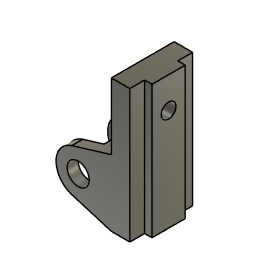
Sectional_Views_Model_Sliding_Block (Autodesk Fusion 360 design; units mm, degrees)
Autodesk Fusion 360 part; units mm, degrees
sketch "Sketch1" plane through (0, 0, 0) normal (0, 1, 0) x (1, 0, 0)
  circle A0 centre (0, 0) radius 15
  line L0 (45, 45) -> (70, 45)
  line L1 (45, -45) -> (45, -135)
  line L2 (45, -135) -> (70, -135)
  line L3 (70, -135) -> (70, 0)
  line L4 (70, 0) -> (70, 45)
  line L5 (45, -135) -> (45, -45)
  line L6 (45, -45) -> (-8.7083, -28.7083)
  line L7 (45, 45) -> (-11.6322, 27.8214)
  line L8 (0, -30) -> (0, -31.3498)
  arc A1 (-8.7083, 28.7083) -> (-8.7083, -28.7083) centre (0, 0) ccw
  dimension "d1" = 60
  dimension "d2" = 30
  dimension "d3" = 70
  dimension "d5" = 25
  dimension "d6" = 180
  constraint coincident A0.centre A1.centre
  constraint concentric A0 A1
  constraint perpendicular L0 L1
  constraint perpendicular L1 L2
  constraint perpendicular L0 L4
  constraint tangent L6 A1
  constraint tangent L7 A1
  constraint coincident L6 L8.end
  constraint coincident L7 A1.start
  measures "d1" diameter of A1
  measures "d2" diameter of A0
  measures "d3" distance of A0.centre L3.end
  measures "d5" distance of L0.end L0.start
  measures "d6" distance of L0.start L1.end
extrude "Extrude1" add sketch "Sketch1" along normal blind 85
sketch "Sketch2" plane through (45, 0, 0) normal (-1, 0, 0) x (0, -1, 0)
  line L0 (0, 45) -> (0, 135)
  line L1 (0, 135) -> (-85, 135)
  line L2 (-85, 135) -> (-85, 45)
  line L3 (-85, 45) -> (0, 45)
sketch "Sketch3" plane through (70, 0, 0) normal (1, 0, 0) x (0, 1, 0)
  line L0 (0, 135) -> (0, -45)
  line L1 (0, -45) -> (85, -45)
  line L2 (85, -45) -> (85, 135)
  line L3 (85, 135) -> (0, 135)
  line L4 (85, -45.5194) -> (85, -45)
  constraint vertical L4
sketch "Sketch4" plane through (70, 0, 0) normal (1, 0, 0) x (0, 1, 0)
  line L0 (20, 135) -> (20, -45)
  line L1 (20, -45) -> (65, -45)
  line L2 (65, -45) -> (65, 135)
  line L3 (65, 135) -> (20, 135)
  constraint vertical L0
  constraint perpendicular L0 L1
  constraint perpendicular L1 L2
  constraint perpendicular L0 L3
extrude "Extrude2" add sketch "Sketch4" along normal blind 10
sketch "Sketch5" plane through (45, 0, 0) normal (-1, 0, 0) x (0, -1, 0)
ref_plane "WorkPlane1" through (45, 0, 135) normal (-1, 0, 0) x (0, -1, 0)
sketch "Sketch6" plane through (45, 0, 0) normal (-1, 0, 0) x (0, -1, 0)
sketch "Sketch7" plane through (45, 0, 0) normal (-1, 0, 0) x (0, -1, 0)
  circle A0 centre (-42.5, 93) radius 25
  dimension "d18" = 50
  measures "d18" diameter of A0
sketch "Sketch8" plane through (45, 0, 0) normal (-1, 0, 0) x (0, -1, 0)
sketch "Sketch9" plane through (45, 0, 0) normal (-1, 0, 0) x (0, -1, 0)
sketch "Sketch10" plane through (45, 0, 0) normal (-1, 0, 0) x (0, -1, 0)
  circle A0 centre (-42.5, 93) radius 10
  dimension "d21" = 20
  measures "d21" diameter of A0
extrude "Extrude3" cut sketch "Sketch10" against normal blind 70
extrude "Extrude4" cut sketch "Sketch7" against normal blind 10
ref_plane "WorkPlane2" through (45, 0, 45) normal (-0.290276, 0, 0.956943) x (0, -1, 0)
sketch "Sketch11" plane through (-8.7083, 0, 28.7083) normal (-0.290276, 0, 0.956943) x (0, -1, 0)
sketch "Sketch12" plane through (0, 0, 0) normal (0, -1, 0) x (1, 0, 0)
  circle A0 centre (0, 0) radius 15
  line L0 (-8.7083, -28.7083) -> (45, -45)
  line L1 (45, -45) -> (70, -45)
  line L2 (70, -45) -> (70, 135)
  line L3 (70, 135) -> (45, 135)
  line L4 (45, 135) -> (45, 45)
  line L5 (45, 45) -> (-8.7083, 28.7083)
  arc A1 (-8.7083, 28.7083) -> (-8.7083, -28.7083) centre (0, 0) ccw
sketch "Sketch13" plane through (70, 0, 0) normal (1, 0, 0) x (0, 1, 0)
sketch "Sketch14" plane through (0, 0, 0) normal (0, -1, 0) x (1, 0, 0)
ref_plane "WorkPlane3" through (45, 0, -45) normal (0, -1, 0) x (1, 0, 0)
sketch "Sketch15" plane through (0, 0, 0) normal (0, -1, 0) x (-1, 0, 0)
ref_plane "WorkPlane4" through (45, 85, -45) normal (0, 1, 0) x (-1, 0, 0)
sketch "Sketch16" plane through (0, 85, 0) normal (0, 1, 0) x (1, 0, 0)
sketch "Sketch17" plane through (-8.7083, 0, 28.7083) normal (-0.290276, 0, 0.956943) x (0, -1, 0)
  line L0 (0, 0) -> (0, 56.1249)
  line L1 (0, 56.1249) -> (-85, 56.1249)
  line L2 (-85, 56.1249) -> (-85, 0)
sketch "Sketch18" plane through (45, 0, 0) normal (-1, 0, 0) x (0, -1, 0)
  line L0 (-85, 45) -> (0, 45)
  line L1 (0, 45) -> (0, 50)
  line L2 (0, 50) -> (-85, 50)
  line L3 (-85, 50) -> (-85, 45)
  constraint horizontal L0
  constraint perpendicular L0 L1
  constraint perpendicular L1 L2
  constraint perpendicular L0 L3
extrude "Extrude5" add sketch "Sketch18" along normal blind 200
sketch "Sketch19" plane through (0, 0, 0) normal (0, -1, 0) x (1, 0, 0)
ref_plane "WorkPlane5" through (-155, 0, 45) normal (0, 0, -1) x (-1, 0, 0)
sketch "Sketch20" plane through (0, 0, 45) normal (0, 0, -1) x (-1, 0, 0)
sketch "Sketch21" plane through (0, 0, 0) normal (0, -1, 0) x (1, 0, 0)
sketch "Sketch22" plane through (0, 85, 0) normal (0, 1, 0) x (-1, 0, 0)
  circle A0 centre (0, 0) radius 15
  line L0 (-45, -45) -> (8.7083, -28.7083)
  arc A1 (8.7083, -28.7083) -> (8.7083, 28.7083) centre (0, 0) ccw
  line L1 (-45, 50) -> (-45, 135)
  line L2 (-45, 135) -> (-70, 135)
  line L3 (-70, 135) -> (-70, -45)
  line L4 (-70, -45) -> (-45, -45)
sketch "Sketch23" plane through (0, 0, 50) normal (0, 0, 1) x (-1, 0, 0)
  line L0 (-45, 0) -> (-45, -85)
  line L1 (-45, -85) -> (155, -85)
  line L2 (155, -85) -> (155, 0)
  line L3 (155, 0) -> (-45, 0)
  line L4 (-20, 0) -> (-20, -85)
  line L5 (-20, -85) -> (164.578, -85)
  line L6 (164.578, -85) -> (164.578, -70)
  line L7 (164.578, -70) -> (-20, -70)
  line L8 (-20, -70) -> (-20, -85)
  line L9 (-20, 0) -> (183.4911, 0)
  line L10 (183.4911, 0) -> (183.4911, -15)
  line L11 (183.4911, -15) -> (-20, -15)
  line L12 (-20, -15) -> (-20, 0)
  dimension "d32" = 15
  dimension "d33" = 15
  constraint coincident L3 L4.start
  constraint coincident L1 L4.end
  constraint perpendicular L1 L4
  constraint horizontal L5
  constraint vertical L6
  constraint horizontal L7
  constraint vertical L8
  constraint horizontal L9
  constraint vertical L10
  constraint horizontal L11
  constraint vertical L12
  measures "d32" distance of L4.end L7.end
  measures "d33" distance of L4.start L11.end
sketch "Sketch24" plane through (0, 0, 0) normal (0, -1, 0) x (1, 0, 0)
extrude "Extrude6" cut sketch "Sketch23" against normal blind 300 contours L2 L4 L7 L11
delete_face "DeleteFace1" 1 faces at (36.6667, 33.3333, 50)
sketch "Sketch25" plane through (70, 0, 0) normal (1, 0, 0) x (0, 1, 0)
sketch "Sketch26" plane through (45, 0, 0) normal (-1, 0, 0) x (0, -1, 0)
sketch "Sketch27" plane through (-8.7083, 0, 28.7083) normal (-0.290276, 0, 0.956943) x (0, -1, 0)
  line L0 (-70, 0) -> (-70, 30)
  line L1 (-70, 30) -> (-15, 30)
  line L2 (-15, 30) -> (-15, 0)
  line L3 (-15, 0) -> (0, 0)
  line L4 (0, 0) -> (0, 56.1249)
  line L5 (0, 56.1249) -> (-85, 56.1249)
  line L6 (-85, 0) -> (-70, 0)
